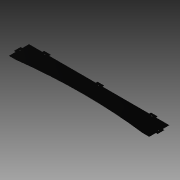
# Autodesk Inventor part: STRUT
Saved by Autodesk Inventor 2013 (Build 170138000, 138)
## iProperties
Created: 2014-03-06
Part Number: STRUT
Material: Generic
Document SubType Name: Modeling
Designer: employee
Density: 1 g/cm^3
Author: employee
Autodesk Inventor part; units mm, degrees
ref_plane "YZ Plane" through (0, 0, 0) normal (1, 0, 0) x (0, 1, 0)
ref_plane "XZ Plane" through (0, 0, 0) normal (0, 1, 0) x (-1, 0, 0)
ref_plane "XY Plane" through (0, 0, 0) normal (0, 0, 1) x (1, 0, 0)
sketch "Sketch1" plane through (0, 0, 0) normal (0, 0, 1) x (1, 0, 0)
  line L0 (-262.5, 75) -> (262.5, 75)
  line L1 (262.5, 75) -> (262.5, 0)
  line L2 (262.5, 0) -> (-262.5, 0)
  line L3 (-262.5, 0) -> (-262.5, 75)
  line L4 (-262.5, 50) -> (-268.977, 50)
  line L5 (-268.977, 50) -> (-268.977, 25)
  line L6 (-268.977, 25) -> (-262.5, 25)
  line L7 (-262.5, 25) -> (-262.5, 50)
  line L8 (-212.5, 75) -> (-187.5, 75)
  line L9 (-187.5, 75) -> (-187.5, 81.477)
  line L10 (-187.5, 81.477) -> (-212.5, 81.477)
  line L11 (-212.5, 81.477) -> (-212.5, 75)
  line L12 (-12.5, 75) -> (12.5, 75)
  line L13 (12.5, 75) -> (12.5, 81.477)
  line L14 (12.5, 81.477) -> (-12.5, 81.477)
  line L15 (-12.5, 81.477) -> (-12.5, 75)
  point P0 (0, 0)
  point P1 (0, 0)
  point P2 (-268.977, 37.5)
  point P3 (-262.5, 37.5)
  point P4 (0, 81.477)
  point P5 (0, 75)
  dimension "d0" = 525
  dimension "d2" = 75
  dimension "d3" = 25
  dimension "d4" = 6.477
  dimension "d5" = 50
  constraints: 32 end point, 8 parallel, 5 midpoint, 4 equal length, 4 horizontal, 4 perpendicular, 3 point on line, 1 coincident, 1 horizontal alignment, 1 vertical alignment
  measures "d0" distance of L1.end L2.end
  measures "d2" distance of L0.end L1.end
  measures "d3" distance of L4.end L5.end
  measures "d4" distance of L4.start L4.end
  measures "d5" distance between parallel lines of L11 L3
extrude "Extrusion1" add sketch "Sketch1" along normal blind 6.477
mirror "Mirror1" about plane through (0, 0, 0) normal (1, 0, 0) of "Extrusion1"
sketch "Sketch2" plane through (0, 0, 6.477) normal (0, 0, 1) x (1, 0, 0)
  line L0 (-187.5, 81.477) -> (-212.5, 81.477) projected
  line L1 (-262.5, 75) -> (-262.5, 50) projected
  line L2 (-268.977, 50) -> (-268.977, 25) projected
  line L3 (12.5, 81.477) -> (-12.5, 81.477) projected
  line L4 (-12.5, 75) -> (-187.5, 75) projected
  line L5 (-260, 39.5) -> (-258.5, 39.5)
  line L6 (-258.5, 39.5) -> (-258.5, 35.5)
  line L7 (-258.5, 35.5) -> (-260, 35.5)
  line L8 (-260, 35.5) -> (-260, 39.5)
  line L9 (-202, 72.5) -> (-198, 72.5)
  line L10 (-198, 72.5) -> (-198, 71)
  line L11 (-198, 71) -> (-202, 71)
  line L12 (-202, 71) -> (-202, 72.5)
  line L13 (-2, 72.5) -> (2, 72.5)
  line L14 (2, 72.5) -> (2, 71)
  line L15 (2, 71) -> (-2, 71)
  line L16 (-2, 71) -> (-2, 72.5)
  point P0 (0, 0)
  point P1 (-268.977, 37.5)
  point P2 (-260, 37.5)
  point P3 (-200, 72.5)
  point P4 (-200, 81.477)
  point P5 (0, 72.5)
  point P6 (0, 81.477)
  dimension "d8" = 4
  dimension "d10" = 1.5
  dimension "d11" = 2.5
  dimension "d13" = 2.5
  constraints: 24 end point, 6 midpoint, 6 parallel, 4 equal length, 3 horizontal, 3 perpendicular, 2 horizontal alignment, 2 vertical alignment
  measures "d8" distance of L5.end L6.end
  measures "d10" distance of L6.end L7.end
  measures "d11" distance between parallel lines of L1 L8
  measures "d13" distance between parallel lines of L4 L9
extrude "Extrusion2" cut sketch "Sketch2" against normal through all
mirror "Mirror2" about plane through (0, 0, 0) normal (1, 0, 0) of "Extrusion2"
sketch "Sketch3" plane through (0, 0, 6.477) normal (0, 0, 1) x (1, 0, 0)
  line L0 (-262.5, 0) -> (262.5, 0) projected
  arc A0 (237.5, 0) -> (-237.5, 0) centre (0, -1872.7083) ccw
  point P0 (0, 0)
  point P1 (0, 15)
  point P2 (0, 0)
  dimension "d16" = 25
  dimension "d17" = 15
  constraints: 3 point on circle, 2 point on line, 1 centre point, 1 midpoint, 1 vertical alignment
  measures "d16" distance of A0.end L0.start
  measures "d17" distance of point (0, 15) point (0, 0)
extrude "Extrusion3" cut sketch "Sketch3" against normal through all
body "Solid1"
